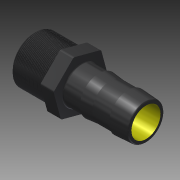
# Autodesk Inventor part: rio grand valley
Saved by Autodesk Inventor 2013 SP2 (Build 170200200, 200)
## iProperties
Created: 2014-07-15
Part Number: rio grand valley
Material: GFRP
Description: HOSE BARB, 1" STRAIGHT (banjo HB100)
Document SubType Name: Modeling
Designer: mrister
Engineer: mrister
Density: 1.75 g/cm^3
Author: mrister
Autodesk Inventor part; units mm, degrees
ref_plane "YZ Plane" through (0, 0, 0) normal (1, 0, 0) x (0, 1, 0)
ref_plane "XZ Plane" through (0, 0, 0) normal (0, 1, 0) x (-1, 0, 0)
ref_plane "XY Plane" through (0, 0, 0) normal (0, 0, 1) x (1, 0, 0)
sketch "Sketch1" plane through (0, 0, 0) normal (0, 0, 1) x (1, 0, 0)
  line L0 (-33.3375, 10.3188) -> (46.0375, 10.3188)
  line L1 (46.0375, 10.3188) -> (46.0375, 12.7)
  line L2 (33.3375, 13.4938) -> (33.3375, 12.7)
  line L3 (33.3375, 12.7) -> (20.6375, 12.7)
  line L4 (12.7, 13.4938) -> (12.7, 12.7)
  line L5 (12.7, 12.7) -> (0, 12.7)
  line L6 (0, 12.7) -> (0, 16.6688)
  line L7 (0, 16.6688) -> (-33.3375, 16.6687)
  line L8 (-33.3375, 16.6687) -> (-33.3375, 10.3188)
  line L9 (0, 12.7) -> (0, 0) construction
  line L10 (12.7, 13.4938) -> (33.3375, 13.4938) construction
  line L11 (33.3375, 12.7) -> (46.0375, 12.7) construction
  line L12 (12.7, 13.4938) -> (20.6375, 12.7)
  line L13 (33.3375, 13.4938) -> (46.0375, 12.7)
  line L14 (-49.2125, 0) -> (61.9125, 0) projected
  dimension "d0" = 10.3187
  dimension "d1" = 16.6687
  dimension "d2" = 12.7
  dimension "d3" = 79.375
  dimension "d4" = 33.3375
  dimension "d5" = 20.6375
  dimension "d6" = 12.7
  dimension "d7" = 13.4938
  constraints: 28 end point, 4 parallel, 4 perpendicular, 3 horizontal, 2 collinear, 1 vertical
  measures "d0" distance from line of L9.end L0
  measures "d1" distance from line of L9.end L7
  measures "d2" vertical distance of L9.end L1.end
  measures "d3" distance of L0.start L0.end
  measures "d4" distance of L6.end L7.end
  measures "d5" distance of L4.start L2.start
  measures "d6" distance of L4.end L5.end
  measures "d7" distance from line of L9.end L10
revolve "Revolution1" add sketch "Sketch1" angle 360 about axis through (-10, 0, 0) along (1, 0, 0)
chamfer "Chamfer1" distance 1.5875 angle 45 2 edges at (-33.3375, -16.6687, 0) (-33.3375, -10.3188, 0)
sketch "Sketch2" plane through (0, 0, 0) normal (0, 0, 1) x (1, 0, 0)
  line L0 (-31.75, 16.6687) -> (0, 16.6687) projected
  line L1 (-55.8405, 16.6687) -> (-55.0467, 16.6687)
  line L2 (-55.0467, 16.6687) -> (-55.4436, 15.875)
  line L3 (-55.4436, 15.875) -> (-55.8405, 16.6687)
  line L4 (-55.4436, 16.6687) -> (-55.4436, 15.875) construction
  point P0 (0, 0)
  dimension "d13" = 0.7937
  constraints: 8 end point, 2 collinear, 1 midpoint, 1 perpendicular, 1 vertical
  measures "d13" distance of L1.start L1.end
coil "Coil1" sketch "Sketch2" operation cut axis through (-10, 0, 0) along (1, 0, 0) pitch 0.9525 turns 160 hand right
sketch "Sketch3" plane through (0, 0, 0) normal (1, 0, 0) x (0, -0.2577648, -0.9662077)
  circle A0 centre (0, 0) radius 12.7 projected
  line L0 (-20.164, 0) -> (-10.082, 17.4625)
  line L1 (-10.082, 17.4625) -> (10.082, 17.4625)
  line L2 (10.082, 17.4625) -> (20.164, 0)
  line L3 (20.164, 0) -> (10.082, -17.4625)
  line L4 (10.082, -17.4625) -> (-10.082, -17.4625)
  line L5 (-10.082, -17.4625) -> (-20.164, 0)
  dimension "d23" = 34.925
  constraints: 12 end point, 1 coincident, 1 horizontal, 13 other
  measures "d23" distance between parallel lines of L3 L0
extrude "Extrusion1" add sketch "Sketch3" against normal blind 9.525
fillet "Fillet1" radius 0.7937 2 edges at (46.0375, -12.7, 0) (0, -12.7, 0)
fillet "Fillet1" radius 1.5875 6 edges at (-4.7625, 19.4712, 5.2401) (-4.7625, 5.1976, 19.4826) (-4.7625, -14.2736, 14.2425) (-4.7625, -19.4712, -5.2401) (-4.7625, -5.1976, -19.4826) (-4.7625, 14.2736, -14.2425)
body "Solid1"
